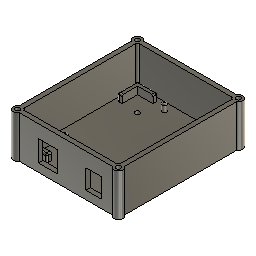
BoitierArduino (Autodesk Fusion 360 design; units mm, degrees)
Autodesk Fusion 360 part; units mm, degrees
note: some values were not read from the file. Set by a fixed rule: which sketch regions a step uses.
sketch "Esquisse1" plane through (0, 0, 0) normal (0, 0, 1) x (1, 0, 0)
  line L0 (0, 0) -> (53.34, 0)
  line L1 (53.34, 0) -> (53.34, 66.04)
  line L2 (48.06, 68.58) -> (15.49, 68.58)
  line L3 (0, 66.04) -> (0, 0)
  line L4 (12.95, 66.04) -> (0, 66.04)
  line L5 (12.95, 66.04) -> (15.49, 68.58)
  line L6 (12.95, 66.04) -> (16.5421, 66.04) construction
  line L7 (50.6, 66.04) -> (53.34, 66.04)
  line L8 (50.6, 66.04) -> (48.06, 68.58)
  line L9 (50.6, 66.04) -> (54.1921, 66.04) construction
  line L10 (0, 0) -> (2.54, 0)
  line L11 (0, 15.24) -> (0, 0)
  line L12 (53.34, 0) -> (50.8, 0)
  line L13 (53.34, 13.97) -> (53.34, 0)
  line L14 (53.34, 66.04) -> (50.6, 66.04)
  line L15 (0, 66.04) -> (12.95, 66.04)
  line L16 (-0.3, 66.04) -> (-0.3, 56.04)
  line L17 (0, 56.04) -> (0, 66.04)
  line L18 (0, 66.04) -> (10, 66.04)
  line L19 (10, 66.34) -> (-0.3, 66.34)
  line L20 (-0.3, 66.34) -> (-0.3, 66.04)
  line L21 (-0.3, 56.04) -> (-3.3, 56.04)
  line L22 (-3.3, 56.04) -> (-3.3, 66.34)
  line L23 (-0.3, 66.34) -> (-0.3, 56.04)
  line L24 (10, 66.34) -> (-0.3, 66.34)
  line L25 (-0.3, 69.34) -> (10, 69.34)
  line L26 (10, 69.34) -> (10, 66.34)
  line L27 (-3.3, 66.34) -> (-3.3, 69.34)
  line L28 (-3.3, 69.34) -> (-0.3, 69.34)
  line L29 (-0.2984, 0.0305) -> (-0.2984, 9.0305)
  line L30 (0, 9) -> (0, 0)
  line L31 (0, 0) -> (9.0015, 0)
  line L32 (9.0015, -0.2695) -> (-0.2984, -0.2695)
  line L33 (-0.2984, -0.2695) -> (-0.2984, 0.0305)
  line L34 (-0.2984, 9.0305) -> (-3.2984, 9.0305)
  line L35 (-3.2984, 9.0305) -> (-3.2984, -0.3)
  line L36 (-0.2984, -0.2695) -> (-0.2984, 9.0305)
  line L37 (9.0015, -0.2695) -> (0.0015, -0.2695)
  line L38 (0, 0) -> (0, 2.7305)
  line L39 (9.0015, -0.2695) -> (-0.2984, -0.2695)
  line L40 (-3.2984, -0.3) -> (-3.2984, -3.2695)
  line L41 (-3.2984, -3.2695) -> (9.0015, -3.2695)
  line L42 (9.0015, -3.2695) -> (9.0015, -0.2695)
  line L43 (53.34, 0) -> (53.34, 33.02)
  line L44 (53.64, 33.02) -> (53.64, 43.02)
  line L45 (53.34, 43.02) -> (53.34, 33.02)
  line L46 (53.64, 33.02) -> (53.64, 23.02)
  line L47 (53.64, 43.02) -> (56.64, 43.02)
  line L48 (56.64, 43.02) -> (56.64, 23.02)
  line L49 (56.64, 23.02) -> (53.64, 23.02)
  line L50 (53.64, 23.02) -> (53.64, 43.02)
  circle A0 centre (45.72, 66.04) radius 1.5
  circle A1 centre (17.78, 66.04) radius 1.5
  circle A2 centre (50.8, 13.97) radius 1.5
  circle A3 centre (2.54, 15.24) radius 1.5
  line L51 (-3.2985, -8.2695) -> (-8.2985, -8.2695)
  line L52 (56.64, 74.34) -> (61.64, 74.34)
  line L53 (-8.2985, -8.2695) -> (61.64, -8.2695)
  line L54 (61.64, -8.2695) -> (61.64, 74.34)
  line L55 (61.64, 74.34) -> (-8.2985, 74.34)
  line L56 (-8.2985, 74.34) -> (-8.2985, -8.2695)
  line L57 (-8.2985, 74.34) -> (-8.2985, 71.34)
  line L58 (-5.2985, 71.34) -> (58.64, 71.34)
  line L59 (-8.2985, -8.2695) -> (-5.2985, -8.2695)
  line L60 (-8.2985, -5.2695) -> (-8.2985, -8.2695)
  line L61 (-5.2985, -5.2695) -> (-5.2985, 71.34)
  line L62 (61.64, -8.2695) -> (58.64, -8.2695)
  line L63 (61.64, -5.2695) -> (61.64, -8.2695)
  line L64 (61.64, 74.34) -> (58.64, 74.34)
  line L65 (61.64, 71.34) -> (61.64, 74.34)
  line L66 (58.64, 71.34) -> (58.64, -5.2695)
  line L67 (-5.2985, -5.2695) -> (58.64, -5.2695)
  line L68 (61.64, 74.34) -> (60.14, 74.34)
  line L69 (60.14, 74.34) -> (60.14, 72.84)
  line L70 (60.14, 72.84) -> (61.64, 72.84)
  line L71 (61.64, 72.84) -> (61.64, 74.34)
  circle A4 centre (60.14, 72.84) radius 3
  line L72 (61.64, -8.2695) -> (60.14, -8.2695)
  line L73 (60.14, -8.2695) -> (60.14, -6.7695)
  line L74 (60.14, -6.7695) -> (61.64, -6.7695)
  line L75 (61.64, -6.7695) -> (61.64, -8.2695)
  circle A5 centre (60.14, -6.7695) radius 3
  line L76 (-8.2985, -8.2695) -> (-6.7985, -8.2695)
  line L77 (-6.7985, -8.2695) -> (-6.7985, -6.7695)
  line L78 (-6.7985, -6.7695) -> (-8.2985, -6.7695)
  line L79 (-8.2985, -6.7695) -> (-8.2985, -8.2695)
  circle A6 centre (-6.7985, -6.7695) radius 3
  line L80 (-8.2985, 74.34) -> (-6.7985, 74.34)
  line L81 (-6.7985, 74.34) -> (-6.7985, 72.84)
  line L82 (-6.7985, 72.84) -> (-8.2985, 72.84)
  line L83 (-8.2985, 72.84) -> (-8.2985, 74.34)
  circle A7 centre (-6.7985, 72.84) radius 3
  dimension "LargeurArduino" = 53.34
  dimension "d5" = 45
  dimension "d8" = 135
  dimension "d9" = 17.78
  dimension "d10" = 7.62
  dimension "d13" = 2.54
  dimension "d14" = 15.24
  dimension "d15" = 2.54
  dimension "d16" = 13.97
  dimension "DistanceMorsArduino" = 0.3
  dimension "d27" = 10
  dimension "d28" = 10.3
  dimension "d29" = 0.3
  dimension "d30" = 3
  dimension "d31" = 10.3
  dimension "d32" = 10.3
  dimension "d33" = 3
  dimension "d34" = 3
  dimension "d35" = 3
  dimension "d36" = 0.3
  dimension "d37" = 9
  dimension "d38" = 9.3
  dimension "d39" = 0.3
  dimension "d40" = 3
  dimension "d41" = 9.3
  dimension "d42" = 9
  dimension "d44" = 12.3
  dimension "d45" = 3
  dimension "d46" = 33.02
  dimension "d47" = 0.3
  dimension "d48" = 10
  dimension "d49" = 0.3
  dimension "d51" = 3
  dimension "d52" = 20
  dimension "d54" = 3
  dimension "d55" = 3
  dimension "d56" = 3
  dimension "d59" = 5
  dimension "d60" = 5
  dimension "d63" = 5
  dimension "EpaisseurBoitier" = 3
  dimension "d65" = 3
  dimension "d66" = 3
  dimension "d67" = 3
  dimension "d68" = 3
  dimension "d69" = 3
  dimension "d70" = 3
  dimension "d71" = 3
  dimension "d72" = 1.5
  dimension "d73" = 1.5
  dimension "d74" = 6
  dimension "d75" = 1.5
  dimension "d76" = 1.5
  dimension "d77" = 6
  dimension "d78" = 1.5
  dimension "d79" = 1.5
  dimension "d80" = 6
  dimension "d81" = 1.5
  dimension "d82" = 1.5
  dimension "d83" = 6
  constraint horizontal L0
  constraint vertical L1
  constraint horizontal L2
  constraint vertical L3
  constraint coincident L0.start L3.end
  constraint horizontal L4
  constraint horizontal L6
  constraint horizontal L7
  constraint horizontal L9
  constraint perpendicular L3 L15
  constraint perpendicular L1 L14
  constraint horizontal L10
  constraint vertical L11
  constraint horizontal L12
  constraint vertical L13
  constraint vertical L16
  constraint vertical L17
  constraint horizontal L18
  constraint horizontal L19
  constraint vertical L20
  constraint horizontal L21
  constraint vertical L22
  constraint vertical L23
  constraint horizontal L24
  constraint horizontal L25
  constraint vertical L26
  constraint vertical L27
  constraint horizontal L28
  constraint vertical L29
  constraint vertical L30
  constraint horizontal L31
  constraint horizontal L32
  constraint vertical L33
  constraint horizontal L34
  constraint vertical L35
  constraint vertical L36
  constraint horizontal L37
  constraint vertical L38
  constraint horizontal L39
  constraint vertical L40
  constraint horizontal L41
  constraint vertical L42
  constraint perpendicular L0 L43
  constraint vertical L44
  constraint vertical L45
  constraint vertical L46
  constraint horizontal L47
  constraint vertical L48
  constraint horizontal L49
  constraint vertical L50
  constraint horizontal L53
  constraint vertical L54
  constraint horizontal L55
  constraint vertical L56
  constraint coincident L56 L57.end
  constraint perpendicular L54 L58
  constraint horizontal L59
  constraint vertical L60
  constraint horizontal L62
  constraint vertical L63
  constraint horizontal L64
  constraint vertical L65
  constraint horizontal L68
  constraint vertical L69
  constraint horizontal L70
  constraint vertical L71
  constraint coincident L69.end L70.start
  constraint horizontal L72
  constraint vertical L73
  constraint horizontal L74
  constraint vertical L75
  constraint coincident L73.end L74.start
  constraint horizontal L76
  constraint vertical L77
  constraint horizontal L78
  constraint vertical L79
  constraint coincident L77.end L78.start
  constraint horizontal L80
  constraint vertical L81
  constraint horizontal L82
  constraint vertical L83
  constraint coincident L81.end L82.start
  measures "LargeurArduino" distance of L0.start L0.end
  measures "d5" angle of L5 L6
  measures "d8" angle of L8 L9
  measures "d9" distance of L3.start A1.centre
  measures "d10" distance of L1.end A0.centre
  measures "d13" distance of L0.start L10.end
  measures "d14" distance of L0.start L11.start
  measures "d15" distance of L0.end L12.end
  measures "d16" distance of L0.end L13.start
  measures "DistanceMorsArduino" distance of L3.start L16.start
  measures "d27" distance of L3.start L17.start
  measures "d28" distance of L16.start L18.end
  measures "d29" distance of L16.start L19.end
  measures "d30" distance of L16.end L21.end
  measures "d31" distance of L16.end L19.end
  measures "d32" distance of L19.start L19.end
  measures "d33" distance of L19.start L25.end
  measures "d34" distance of L19.end L22.end
  measures "d35" distance of L19.end L25.start
  measures "d36" distance of L0.start L29.start
  measures "d37" distance of L0.start L30.start
  measures "d38" distance of L29.start L31.end
  measures "d39" distance of L29.start L32.end
  measures "d40" distance of L29.end L34.end
  measures "d41" distance of L29.end L32.end
  measures "d42" distance of L32.start L37.end
  measures "d44" distance of L32.start L35.end
  measures "d45" distance of L32.start L41.end
  measures "d46" distance of L0.end L43.end
  measures "d47" distance of L43.end L44.start
  measures "d48" distance of L43.end L45.start
  measures "d49" distance of L43.end L44.start
  measures "d51" distance of L44.end L47.end
  measures "d52" distance of L44.end L46.end
  measures "d54" diameter of A1
  measures "d55" diameter of A2
  measures "d56" diameter of A3
  measures "d59" distance of L40.end L51.start
  measures "d60" distance of L51.start L51.end
  measures "d63" distance of L52.start L52.end
  measures "EpaisseurBoitier" distance of L55.end L57.end
  measures "d65" distance of L57.end L58.start
  measures "d66" distance of L51.end L59.end
  measures "d67" distance of L51.end L60.start
  measures "d68" distance of L53.end L62.end
  measures "d69" distance of L53.end L63.start
  measures "d70" distance of L52.end L64.end
  measures "d71" distance of L52.end L65.start
  measures "d72" distance of L52.end L68.end
  measures "d73" distance of L52.end L70.end
  measures "d74" diameter of A4
  measures "d75" distance of L53.end L72.end
  measures "d76" distance of L53.end L74.end
  measures "d77" diameter of A5
  measures "d78" distance of L51.end L76.end
  measures "d79" distance of L51.end L78.end
  measures "d80" diameter of A6
  measures "d81" distance of L55.end L80.end
  measures "d82" distance of L55.end L82.end
  measures "d83" diameter of A7
sketch "Esquisse2" plane through (0, 0, 0) normal (0, 0, 1) x (1, 0, 0)
extrude "Extrusion1" add sketch "Esquisse1" against normal blind 3 contours L0 L1 L2 L3 L4 L5 L7 L8 L10 L11 L12 L13 L14 L15 L17 L18 L30 L31 L38 L43 L45 | L16 L19 L20 L21 L22 L23 L24 L25 L26 L27 L28 | L29 L32 L33 L34 L35 L36 L37 L39 L40 L41 L42 | L44 L46 L47 L48 L49 L50 | A0 | A1 | A2 | A3 | L51 L53 L56 L59 L60 L76 L79 A6 | L51 L53 L56 L59 L60 L61 L67 L77 L78 A6 | L51 L53 L56 L59 L60 L76 L77 L78 L79 | L51 L53 L67 A5 A6 | L56 L61 A6 A7 | L53 L54 L62 L63 L66 L67 L73 L74 A5 | L53 L54 L62 L63 L72 L75 A5 | L55 L56 L57 L80 L83 A7 | L55 L56 L57 L58 L61 L81 L82 A7 | L61 L67 A6 | L58 L61 L66 L67 A4 A5 A6 A7 | L66 L67 A5 | L52 L55 L58 A4 A7 | L58 L61 A7 | L53 L54 L62 L63 L72 L73 L74 L75 | L54 L66 A4 A5 | L55 L56 L57 L80 L81 L82 L83 | L58 L66 A4 | L52 L54 L55 L58 L64 L65 L66 L69 L70 A4 | L52 L54 L55 L64 L65 L68 L71 A4 | L52 L54 L55 L64 L65 L68 L69 L70 L71
extrude "Extrusion2" add sketch "Esquisse1" along normal blind 5 contours L16 L19 L20 L21 L22 L23 L24 L25 L26 L27 L28 | L29 L32 L33 L34 L35 L36 L37 L39 L40 L41 L42 | L44 L46 L47 L48 L49 L50
extrude "Extrusion3" add sketch "Esquisse1" along normal blind 25 contours L51 L53 L56 L59 L60 L76 L79 A6 | L51 L53 L56 L59 L60 L61 L67 L77 L78 A6 | L51 L53 L56 L59 L60 L76 L77 L78 L79 | L51 L53 L67 A5 A6 | L56 L61 A6 A7 | L53 L54 L62 L63 L66 L67 L73 L74 A5 | L53 L54 L62 L63 L72 L75 A5 | L55 L56 L57 L80 L83 A7 | L55 L56 L57 L58 L61 L81 L82 A7 | L61 L67 A6 | L66 L67 A5 | L52 L55 L58 A4 A7 | L58 L61 A7 | L53 L54 L62 L63 L72 L73 L74 L75 | L54 L66 A4 A5 | L55 L56 L57 L80 L81 L82 L83 | L58 L66 A4 | L52 L54 L55 L58 L64 L65 L66 L69 L70 A4 | L52 L54 L55 L64 L65 L68 L71 A4 | L52 L54 L55 L64 L65 L68 L69 L70 L71
extrude "Extrusion4" add sketch "Esquisse1" along normal blind 5 contours A0 | A1 | A2 | A3
fillet "Congé1" radius 1 1 edges at (16.3815, 65.4976, 5)
fillet "Congé2" radius 1 1 edges at (44.3215, 65.4976, 5)
fillet "Congé3" radius 1 1 edges at (49.4015, 13.4276, 5)
fillet "Congé4" radius 1 1 edges at (1.1415, 14.6976, 5)
fillet "Congé5" radius 1 1 edges at (-3.3, 62.69, 5)
fillet "Congé6" radius 1 4 edges at (3.85, 69.34, 5) (-3.0071, 69.34, 4.7071) (-3.3, 69.34, 2) (56.64, 33.02, 5)
fillet "Congé7" radius 1 2 edges at (2.8515, -3.2695, 5) (-3.2984, 2.8805, 5)
fillet "Congé8" radius 1 18 edges at (56.64, 23.02, 2) (56.3471, 23.02, 4.7071) (54.64, 23.02, 5) (56.64, 43.02, 2) (56.3471, 43.02, 4.7071) (54.64, 43.02, 5) (-3.3, 56.04, 2) (-3.0071, 56.04, 4.7071) (-1.3, 56.04, 5) (10, 67.34, 5) (10, 69.0471, 4.7071) (10, 69.34, 2) (-1.2984, 9.0305, 5) (-3.0056, 9.0305, 4.7071) (-3.2984, 9.0305, 2) (9.0015, -3.2695, 2) (9.0015, -2.9766, 4.7071) (9.0015, -1.2695, 5)
sketch "Esquisse3" plane through (0, 0, 0) normal (0, 0, 1) x (1, 0, 0)
  line L0 (0, 0) -> (9.3, 0)
  line L1 (9.3, 0) -> (20.35, 0)
  line L2 (20.35, 0) -> (20.35, 12.9937)
  line L3 (20.35, 12.9937) -> (9.3, 12.9937)
  line L4 (9.3, 12.9937) -> (9.3, 0)
  line L5 (53, 0) -> (49.82, 0)
  line L6 (49.82, 0) -> (39.84, 0)
  line L7 (39.84, 0) -> (50, 0)
  line L8 (50, 0) -> (50, 8)
  line L9 (50, 8) -> (39.84, 8)
  line L10 (39.84, 8) -> (39.84, 0)
  dimension "d108" = 9.3
  dimension "d109" = 11.05
  dimension "d110" = 3.18
  dimension "d111" = 9.98
  constraint coincident L0.start origin
  constraint horizontal L0
  constraint horizontal L1
  constraint vertical L2
  constraint horizontal L3
  constraint vertical L4
  constraint horizontal L5
  constraint parallel L5 L6
  constraint horizontal L7
  constraint vertical L8
  constraint horizontal L9
  constraint vertical L10
  measures "d108" distance of L0.start L0.end
  measures "d109" distance of L0.end L1.end
  measures "d110" distance of L5.start L5.end
  measures "d111" distance of L5.end L6.end
extrude "Extrusion5" add sketch "Esquisse3" along normal blind 15.15 contours L1 L2 L3 L4
extrude "Extrusion6" add sketch "Esquisse3" along normal blind 13.45 contours L5 L6 L7 L8 L9 L10
sketch "Esquisse4" plane through (0, 0, 0) normal (0, 0, 1) x (1, 0, 0)
  line L0 (50, 0) -> (50, -8.5293)
  line L1 (20, 0) -> (20, -9)
  line L2 (9, 0) -> (9, -9)
  line L3 (9, -9) -> (20, -9)
  line L4 (40, 0) -> (40, -9)
  line L5 (40, -9) -> (50, -9)
  line L6 (50, -9) -> (50, -8.5293)
  constraint vertical L0
  constraint parallel L0 L1
  constraint vertical L2
  constraint perpendicular L1 L3
  constraint vertical L4
  constraint perpendicular L4 L5
sketch "Esquisse5" plane through (0, -8.2695, 0) normal (0, -1, 0) x (1, 0, 0)
  line L0 (-4.2004, 25) -> (-4.2004, -3)
  line L1 (-4.2004, -3) -> (57.5419, -3)
  line L2 (57.5419, -3) -> (57.5419, 25)
  line L3 (57.5419, 25) -> (-4.2004, 25)
  line L4 (50, 0) -> (40, 0)
  line L5 (40, 0) -> (50, 0)
  line L6 (50, 0) -> (50, 2.45)
  line L7 (50, 2.45) -> (40, 2.45)
  line L8 (40, 2.45) -> (40, 0)
  line L9 (40, 2.45) -> (50.0667, 2.45)
  line L10 (50.0667, 2.45) -> (50.0667, 15.45)
  line L11 (50.0667, 15.45) -> (40, 15.45)
  line L12 (40, 15.45) -> (40, 2.45)
  line L13 (8.4706, -0.037) -> (21, -0.037)
  line L14 (21, -0.037) -> (21, 2.413)
  line L15 (21, 2.413) -> (8.4706, 2.413)
  line L16 (8.4706, 2.413) -> (8.4706, -0.037)
  line L17 (8.4706, 2.413) -> (21.0631, 2.413)
  line L18 (21.0631, 2.413) -> (21.0631, 16.413)
  line L19 (21.0631, 16.413) -> (8.4706, 16.413)
  line L20 (8.4706, 16.413) -> (8.4706, 2.413)
  dimension "d116" = 2.45
  dimension "d117" = 13
  dimension "d118" = 2.45
  dimension "d119" = 14
  constraint parallel L1 L4
  constraint horizontal L5
  constraint vertical L6
  constraint horizontal L7
  constraint vertical L8
  constraint horizontal L9
  constraint vertical L10
  constraint horizontal L11
  constraint vertical L12
  constraint horizontal L13
  constraint vertical L14
  constraint horizontal L15
  constraint vertical L16
  constraint horizontal L17
  constraint vertical L18
  constraint horizontal L19
  constraint vertical L20
  measures "d116" distance of L4.end L7.end
  measures "d117" distance of L7.end L11.end
  measures "d118" distance of L13.start L15.end
  measures "d119" distance of L15.end L19.end
extrude "Extrusion7" cut sketch "Esquisse5" against normal blind 4 contours L7 L9 L10 L11 L12 | L15 L17 L18 L19 L20
extrude "Extrusion8" cut 1 faces at (12.9833, 8.6625, 15.15) along direction (0, 0, -1) blind 15
extrude "Extrusion9" cut 1 faces at (12.9833, 8.6625, 0.15) along direction (0, 0, -1) blind 0.15
extrude "Extrusion10" cut 1 faces at (46.6133, 2.6667, 13.45) along direction (0, 0, -1) blind 13.45
sketch "Esquisse6" plane through (0, 0, 0) normal (0, 0, 1) x (1, 0, 0)
  line L0 (0, 66) -> (53.34, 66)
  line L1 (53.34, 66) -> (53.34, -0.04)
  line L2 (53.34, -0.04) -> (0, -0.04)
  line L3 (0, -0.04) -> (0, 66)
  line L4 (53.34, 66) -> (43.34, 66)
  line L5 (43.34, 66) -> (43.34, 56)
  line L6 (43.34, 56) -> (53.34, 56)
  line L7 (53.34, 56) -> (53.34, 66)
  line L8 (0, 66) -> (10, 66)
  line L9 (10, 66) -> (10, 56)
  line L10 (10, 56) -> (0, 56)
  line L11 (0, 56) -> (0, 66)
  line L12 (53.34, -0.04) -> (43.34, -0.04)
  line L13 (43.34, -0.04) -> (43.34, 9.96)
  line L14 (43.34, 9.96) -> (53.34, 9.96)
  line L15 (53.34, 9.96) -> (53.34, -0.04)
  line L16 (0, 0) -> (10, 0)
  line L17 (10, 0) -> (10, 10)
  line L18 (10, 10) -> (0, 10)
  line L19 (0, 10) -> (0, 0)
  circle A0 centre (10, 10) radius 1.5
  circle A1 centre (43.34, 9.96) radius 1.5
  circle A2 centre (10, 56) radius 1.5
  circle A3 centre (43.34, 56) radius 1.5
  dimension "d128" = 53.34
  dimension "d129" = 66.04
  dimension "d130" = 10
  dimension "d131" = 10
  dimension "d132" = 10
  dimension "d133" = 10
  dimension "d134" = 10
  dimension "d135" = 10
  dimension "d136" = 10
  dimension "d137" = 10
  dimension "d139" = 3
  dimension "d140" = 3
  dimension "d141" = 3
  constraint horizontal L0
  constraint vertical L1
  constraint horizontal L2
  constraint vertical L3
  constraint horizontal L4
  constraint vertical L5
  constraint horizontal L6
  constraint vertical L7
  constraint horizontal L8
  constraint vertical L9
  constraint horizontal L10
  constraint vertical L11
  constraint horizontal L12
  constraint vertical L13
  constraint horizontal L14
  constraint vertical L15
  constraint horizontal L16
  constraint vertical L17
  constraint horizontal L18
  constraint vertical L19
  constraint coincident L16.start L19.end
  constraint coincident L17.end L18.start
  constraint coincident L13.end L14.start
  constraint coincident L9.end L10.start
  constraint coincident L5.end L6.start
  measures "d128" distance of L0.start L0.end
  measures "d129" distance of L0.start L2.end
  measures "d130" distance of L0.end L4.end
  measures "d131" distance of L0.end L6.end
  measures "d132" distance of L0.start L8.end
  measures "d133" distance of L0.start L10.end
  measures "d134" distance of L1.end L12.end
  measures "d135" distance of L1.end L14.end
  measures "d136" distance of L16.start L16.end
  measures "d137" distance of L16.start L18.end
  measures "d139" diameter of A1
  measures "d140" diameter of A2
  measures "d141" diameter of A3
extrude "Extrusion11" cut sketch "Esquisse6" against normal blind 9 contours L9 L10 A2 | L9 L10 A2
extrude "Extrusion12" cut sketch "Esquisse6" against normal blind 7 contours L5 L6 A3 | L5 L6 A3
extrude "Extrusion13" cut sketch "Esquisse6" against normal blind 6 contours L17 L18 A0 | L17 L18 A0
extrude "Extrusion14" cut sketch "Esquisse6" against normal blind 8 contours L13 L14 A1 | L13 L14 A1
sketch "Esquisse7" plane through (0, 0, 25) normal (0, 0, 1) x (-1, 0, 0)
  line L0 (-57.5419, 5.2695) -> (4.2004, 5.2695)
  arc A0 (4.2004, 5.2695) -> (5.2985, 4.1714) centre (6.7985, 6.7695) ccw
  line L1 (5.2985, 4.1714) -> (5.2985, -70.2419)
  arc A1 (5.2985, -70.2419) -> (4.2004, -71.34) centre (6.7985, -72.84) ccw
  line L2 (4.2004, -71.34) -> (-57.5419, -71.34)
  arc A2 (-57.5419, -71.34) -> (-58.64, -70.2419) centre (-60.14, -72.84) ccw
  line L3 (-58.64, -70.2419) -> (-58.64, 4.1714)
  arc A3 (-58.64, 4.1714) -> (-57.5419, 5.2695) centre (-60.14, 6.7695) ccw
  line L4 (-57.5419, -74.34) -> (4.2004, -74.34)
  arc A4 (4.2004, -74.34) -> (8.2985, -70.2419) centre (6.7985, -72.84) ccw
  line L5 (8.2985, -70.2419) -> (8.2985, 4.1714)
  arc A5 (8.2985, 4.1714) -> (4.2004, 8.2695) centre (6.7985, 6.7695) ccw
  line L6 (4.2004, 8.2695) -> (-57.5419, 8.2695)
  arc A6 (-57.5419, 8.2695) -> (-61.64, 4.1714) centre (-60.14, 6.7695) ccw
  line L7 (-61.64, 4.1714) -> (-61.64, -70.2419)
  arc A7 (-61.64, -70.2419) -> (-57.5419, -74.34) centre (-60.14, -72.84) ccw
  circle A8 centre (6.7985, -72.84) radius 1.5
  circle A9 centre (-60.14, -72.84) radius 1.5
  circle A10 centre (-60.14, 6.7695) radius 1.5
  circle A11 centre (6.7985, 6.7695) radius 1.5
  dimension "d150" = 3
  dimension "d151" = 3
  dimension "d152" = 3
  dimension "d153" = 3
  constraint concentric A1 A8
  constraint concentric A2 A9
  constraint concentric A3 A10
  constraint concentric A0 A11
  measures "d150" diameter of A8
  measures "d151" diameter of A9
  measures "d152" diameter of A10
  measures "d153" diameter of A11
hole "Perçage1" at (60.14, -6.7695, 25) at (-6.7985, -6.7695, 25) at (60.14, 72.84, 25) at (-6.7985, 72.84, 25) direction (0, 0, -1) diameter 3 depth 20 tip angle 118
sketch "Esquisse8" plane through (0, 0, 0) normal (0, 0, 1) x (1, 0, 0)
component "BoitierArduino" placed x (1, 0, 0) y (0, 1, 0) z (0, 0, 1) at (0, 0, 0)
equation "LongueurArduino = 68.58 mm"
equation "DiamètreArduino = 3.2 mm"
equation "LargeurBoitier = 90 mm"
equation "LongueurBoitier = 100 mm"
equation "EpaisseurMors = 3 mm"
equation "d29 = DistanceMorsArduino"
equation "d30 = EpaisseurMors"
equation "d33 = EpaisseurMors"
equation "d36 = DistanceMorsArduino"
equation "d39 = DistanceMorsArduino"
equation "d40 = EpaisseurMors"
equation "d45 = EpaisseurMors"
equation "d47 = DistanceMorsArduino"
equation "d49 = DistanceMorsArduino"
equation "d51 = EpaisseurMors"
equation "DiamètreMors = 3 mm"
equation "d54 = DiamètreMors"
equation "d55 = DiamètreMors"
equation "d56 = DiamètreMors"
equation "DistanceMorsBoitier = 5 mm"
equation "d59 = DistanceMorsBoitier"
equation "d60 = DistanceMorsBoitier"
equation "d63 = DistanceMorsBoitier"
equation "d65 = EpaisseurBoitier"
equation "d66 = EpaisseurBoitier"
equation "d67 = EpaisseurBoitier"
equation "d68 = EpaisseurBoitier"
equation "d69 = EpaisseurBoitier"
equation "d70 = EpaisseurBoitier"
equation "d71 = EpaisseurBoitier"
equation "d72 = EpaisseurBoitier / 2"
equation "d73 = EpaisseurBoitier / 2"
equation "d74 = EpaisseurBoitier * 2"
equation "d75 = EpaisseurBoitier / 2"
equation "d76 = EpaisseurBoitier / 2"
equation "d77 = EpaisseurBoitier * 2"
equation "d78 = EpaisseurBoitier / 2"
equation "d79 = EpaisseurBoitier / 2"
equation "d80 = EpaisseurBoitier * 2"
equation "d81 = EpaisseurBoitier / 2"
equation "d82 = EpaisseurBoitier / 2"
equation "d83 = EpaisseurBoitier * 2"
equation "d84 = -EpaisseurBoitier"
equation "HauteurMors = 5 mm"
equation "HauteurBoitier = 25 mm"
equation "d90 = HauteurMors"
equation "CongéMors = 1 mm"
equation "d95 = CongéMors"
equation "d97 = CongéMors"
equation "d99 = CongéMors"
equation "d101 = CongéMors"
equation "d103 = CongéMors"
equation "d105 = CongéMors"
equation "d107 = CongéMors"
equation "d128 = LargeurArduino"
equation "d129 = LongueurArduino - 2.54 mm"
equation "DiamètreVis = 3 mm"
equation "d139 = DiamètreVis"
equation "d140 = DiamètreVis"
equation "d141 = DiamètreVis"
equation "d150 = DiamètreVis"
equation "d151 = DiamètreVis"
equation "d152 = DiamètreVis"
equation "d153 = DiamètreVis"
equation "d155 = DiamètreVis"
